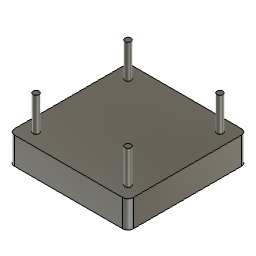
ir_camera_holder (Autodesk Fusion 360 design; units mm, degrees)
Autodesk Fusion 360 part; units mm, degrees
sketch "Sketch1" plane through (0, 0, 0) normal (0, 0, 1) x (1, 0, 0)
  line L0 (-20, 22) -> (20, 22)
  line L1 (22, 20) -> (22, -20)
  line L2 (20, -22) -> (-20, -22)
  line L3 (-22, -20) -> (-22, 20)
  arc A0 (-20, 22) -> (-22, 20) centre (-20, 20) ccw
  arc A1 (22, 20) -> (20, 22) centre (20, 20) ccw
  arc A2 (20, -22) -> (22, -20) centre (20, -20) ccw
  arc A3 (-22, -20) -> (-20, -22) centre (-20, -20) ccw
  point P0 (-22, 22)
  point P1 (22, 22)
  point P2 (-22, -22)
  dimension "d1" = 44
  dimension "d2" = 44
  dimension "d3" = 2
  constraint horizontal L0
  constraint vertical L1
  constraint horizontal L2
  constraint vertical L3
  constraint coincident P0 L0
  constraint coincident P0 L3
  constraint tangent L0 A0
  constraint tangent L3 A0
  constraint coincident P1 L0
  constraint coincident P1 L1
  constraint tangent L0 A1
  constraint tangent L1 A1
  constraint equal A0 A1
  constraint tangent L1 A2
  constraint tangent L2 A2
  constraint equal A0 A2
  constraint coincident P2 L2
  constraint coincident P2 L3
  constraint tangent L2 A3
  constraint tangent L3 A3
  constraint equal A0 A3
  measures "d1" distance of P0 P1
  measures "d2" distance of P0 P2
  measures "d3" radius of A0
extrude "Extrude1" add sketch "Sketch1" along normal mid plane 10
sketch "Sketch2" plane through (0, 0, 5) normal (0, 0, 1) x (-1, 0, 0)
  arc A0 (20, -22) -> (22, -20) centre (20, -20) ccw
  line L0 (22, -20) -> (22, 20)
  arc A1 (22, 20) -> (20, 22) centre (20, 20) ccw
  line L1 (20, 22) -> (-20, 22)
  arc A2 (-20, 22) -> (-22, 20) centre (-20, 20) ccw
  line L2 (-22, 20) -> (-22, -20)
  arc A3 (-22, -20) -> (-20, -22) centre (-20, -20) ccw
  line L3 (-20, -22) -> (20, -22)
  circle A4 centre (17, -17) radius 1.125
  circle A5 centre (-17, -17) radius 1.125
  circle A6 centre (17, 17) radius 1.125
  circle A7 centre (-17, 17) radius 1.125
  dimension "d6" = 34
  dimension "d7" = 34
  dimension "d8" = 2.25
  dimension "d9" = 2.25
  dimension "d10" = 2.25
  dimension "d11" = 2.25
  measures "d6" distance of A4.centre A5.centre
  measures "d7" distance of A5.centre A7.centre
  measures "d8" diameter of A4
  measures "d9" diameter of A5
  measures "d10" diameter of A6
  measures "d11" diameter of A7
extrude "Extrude2" add sketch "Sketch2" along normal blind 12.5 contours A4 | A5 | A6 | A7
